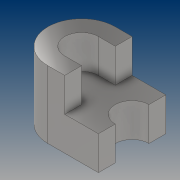
# Autodesk Inventor part: 29
Saved by Autodesk Inventor 2020.2 (Build 242310000, 310)
## iProperties
Created: 2020-09-17
Part Number: 29
Material: 鋼、碳鋼
Document SubType Name: Modeling
Designer: user
Density: 7.85 g/cm^3
Appearance: 半拋光
Mass: 367.769 g
Surface Area: 99.1239 cm^2
Volume: 46.8496 cm^3
Author: user
Autodesk Inventor part; units mm, degrees
ref_plane "YZ Plane" through (0, 0, 0) normal (1, 0, 0) x (0, 1, 0)
ref_plane "XZ Plane" through (0, 0, 0) normal (0, 1, 0) x (-1, 0, 0)
ref_plane "XY Plane" through (0, 0, 0) normal (0, 0, 1) x (1, 0, 0)
sketch "草圖1" plane through (0, 0, 0) normal (0, 1, 0) x (-1, 0, 0)
  circle A0 centre (0, 0) radius 20
  line L0 (0, -20) -> (-30, -20)
  line L1 (-30, -20) -> (-30, 20)
  line L2 (-30, 20) -> (0, 20)
  line L3 (0, 20) -> (0, -20)
  point P0 (0, 20)
  dimension "d0" = 40
  dimension "d1" = 30
  constraints: 8 end point, 3 horizontal, 2 parallel, 1 coincident, 1 perpendicular, 3 other
  measures "d1" distance from line of L1 point (0, 0)
extrude "擠出1" add sketch "草圖1" along normal blind 40
sketch "草圖2" plane through (0, 40, 0) normal (0, 1, 0) x (1, 0, 0)
  line L0 (30, -20) -> (0, -20) projected
  arc A0 (0, 20) -> (0, -20) centre (0, 0) ccw projected
  line L1 (0, 20) -> (30, 20) projected
  line L2 (30, 20) -> (30, -20) projected
  line L3 (10, 20) -> (30, 20)
  line L4 (30, 20) -> (30, -20)
  line L5 (30, -20) -> (10, -20)
  line L6 (10, -20) -> (10, 20)
  line L7 (30, -20) -> (30, 20) projected
  line L8 (30, 20) -> (0, 20) projected
  line L9 (0, -20) -> (30, -20) projected
  line L10 (0, 10) -> (10, 10)
  line L11 (10, 10) -> (10, -10)
  line L12 (10, -10) -> (0, -10)
  line L13 (0, -10) -> (0, 10)
  circle A1 centre (0, 0) radius 10
  point P0 (10, 0)
  point P1 (0, -10)
  dimension "d4" = 20
  dimension "d5" = 20
  dimension "d6" = 10
  constraints: 16 end point, 4 parallel, 3 collinear, 2 horizontal, 2 midpoint, 2 perpendicular, 1 centre point, 1 coincident, 1 tangent
  measures "d4" distance between parallel lines of L2 L6
  measures "d5" distance of L12.end L10.start
  measures "d6" distance of L10.start L10.end
extrude "擠出2" cut sketch "草圖2" against normal blind 20 contours L0 L6 L1 L2 | L12 A1 L6 | A1 L10 L6 | A1 L13 | A1 L13
sketch "草圖3" plane through (0, 20, 0) normal (0, 1, 0) x (1, 0, 0)
  line L0 (10, 20) -> (10, 10) projected
  line L1 (10, 10) -> (0, 10) projected
  arc A0 (0, 10) -> (0, -10) centre (0, 0) ccw projected
  line L2 (0, -10) -> (10, -10) projected
  line L3 (10, -10) -> (10, -20) projected
  line L4 (30, -20) -> (10, -20) projected
  line L5 (30, 20) -> (30, -20) projected
  line L6 (10, 20) -> (30, 20) projected
  line L7 (0, 20) -> (10, 20) projected
  arc A1 (0, 20) -> (0, -20) centre (0, 0) ccw projected
  line L8 (10, -20) -> (0, -20) projected
  circle A2 centre (30, 0) radius 10
  dimension "d9" = 20
  constraints: 1 centre point, 1 midpoint
  measures "d9" diameter of A2
extrude "擠出3" cut sketch "草圖3" against normal through all contours A2 L5 | L5 A2
